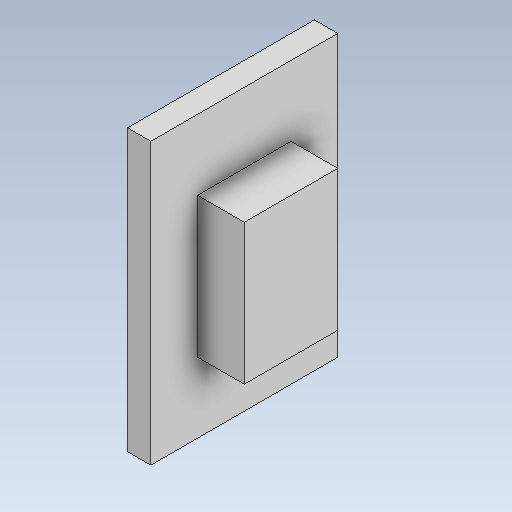
# Autodesk Inventor part: slider
Saved by Autodesk Inventor 2020 (Build 240168000, 168)
## iProperties
Created: 2021-07-04
Part Number: slider
Material: Generic
Document SubType Name: Modeling
Designer: pc
Density: 1 g/cm^3
Appearance: Default
Mass: 294.967 g
Surface Area: 438.709 cm^2
Volume: 294.967 cm^3
Author: pc
Autodesk Inventor part; units mm, degrees
ref_plane "YZ Plane" through (0, 0, 0) normal (1, 0, 0) x (0, 1, 0)
ref_plane "XZ Plane" through (0, 0, 0) normal (0, 1, 0) x (-1, 0, 0)
ref_plane "XY Plane" through (0, 0, 0) normal (0, 0, 1) x (1, 0, 0)
sketch "Sketch1" plane through (0, 0, 0) normal (1, 0, 0) x (0, 1, 0)
  line L0 (9.9359, 10.4879) -> (-142.4641, 10.4879)
  line L1 (-142.4641, 10.4879) -> (-142.4641, -91.1121)
  line L2 (-142.4641, -91.1121) -> (9.9359, -91.1121)
  line L3 (9.9359, -91.1121) -> (9.9359, 10.4879)
  point P0 (0, 0)
  dimension "d0" = 152.4
  dimension "d1" = 101.6
  constraints: 8 end point, 2 parallel, 1 horizontal, 1 perpendicular
  measures "d0" distance of L2.end L1.end
  measures "d1" distance of L1.end L0.end
extrude "Extrusion1" add sketch "Sketch1" along normal blind 12.7
sketch "Sketch2" plane through (12.7, 0, 0) normal (1, 0, 0) x (0, 0, -1)
  line L0 (14.9121, -28.1641) -> (65.7121, -28.1641)
  line L1 (65.7121, -28.1641) -> (65.7121, -104.3641)
  line L2 (65.7121, -104.3641) -> (14.9121, -104.3641)
  line L3 (14.9121, -104.3641) -> (14.9121, -28.1641)
  line L4 (91.1121, -142.4641) -> (91.1121, 9.9359) projected
  line L5 (91.1121, 9.9359) -> (-10.4879, 9.9359) projected
  point P0 (0, 0)
  dimension "d4" = 50.8
  dimension "d5" = 76.2
  dimension "d6" = 25.4
  dimension "d7" = 38.1
  constraints: 8 end point, 2 parallel, 1 horizontal, 1 perpendicular
  measures "d4" distance of L1.end L2.end
  measures "d5" distance of L0.end L1.end
  measures "d6" distance between parallel lines of L1 L4
  measures "d7" distance between parallel lines of L5 L0
extrude "Extrusion2" add sketch "Sketch2" along normal blind 25.4
body "Solid1"
